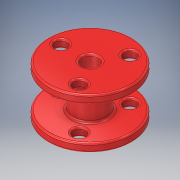
# Autodesk Inventor part: Connecting Rod Hub
Saved by Autodesk Inventor 2017 (Build 210142000, 142)
## iProperties
Created: 2020-01-12
Part Number: Connecting Rod Hub
Material: Stainless Steel
Document SubType Name: Modeling
Designer: Admin
Density: 8 g/cm^3
Appearance: Light Red
Mass: 5.65044 g
Surface Area: 10.6206 cm^2
Volume: 0.706304 cm^3
Author: Admin
Autodesk Inventor part; units mm, degrees
ref_plane "YZ Plane" through (0, 0, 0) normal (1, 0, 0) x (0, 1, 0)
ref_plane "XZ Plane" through (0, 0, 0) normal (0, 1, 0) x (-1, 0, 0)
ref_plane "XY Plane" through (0, 0, 0) normal (0, 0, 1) x (1, 0, 0)
sketch "Sketch1" plane through (0, 0, 0) normal (0, 1, 0) x (-1, 0, 0)
  circle A0 centre (0, 0) radius 3.175
  dimension "d0" = 6.35
  constraints: 1 centre point, 1 coincident
  measures "d0" diameter of A0
extrude "Extrusion1" add sketch "Sketch1" along normal mid plane 6.35
sketch "Sketch2" plane through (0, 3.175, 0) normal (0, 1, 0) x (1, 0, 0)
  circle A0 centre (0, 0) radius 7.9375
  dimension "d3" = 15.875
  constraints: 1 centre point, 1 coincident
  measures "d3" diameter of A0
extrude "Extrusion2" add sketch "Sketch2" along normal blind 1.5875
sketch "Sketch3" plane through (0, -3.175, 0) normal (0, -1, 0) x (1, 0, 0)
  circle A0 centre (0, 0) radius 7.9375
  dimension "d6" = 15.875
  constraints: 1 centre point, 1 coincident
  measures "d6" diameter of A0
extrude "Extrusion3" add sketch "Sketch3" along normal blind 1.5875
sketch "Sketch4" plane through (0, 4.7625, 0) normal (0, 1, 0) x (1, 0, 0)
  circle A0 centre (0, 0) radius 1.5875
  dimension "d9" = 3.175
  constraints: 1 centre point, 1 coincident
  measures "d9" diameter of A0
extrude "Extrusion4" cut sketch "Sketch4" against normal blind 25.4
sketch "Sketch5" plane through (0, 4.7625, 0) normal (0, 1, 0) x (1, 0, 0)
  circle A0 centre (-5.5563, 0) radius 1.1906
  circle A1 centre (2.7781, -4.8119) radius 1.1906
  circle A2 centre (2.7781, 4.8119) radius 1.1906
  point P0 (0, 0)
  dimension "d12" = 2.3813
  dimension "d13" = 0
  dimension "d14" = 5.5563
  dimension "d17" = 360
  constraints: 3 centre point, 7 other
  measures "d12" diameter of A0
  measures "d13" vertical distance of point (0, 0) A0.centre
  measures "d14" distance of point (0, 0) A0.centre
extrude "Extrusion5" cut sketch "Sketch5" against normal blind 25.4
fillet "Fillet1" radius 0.3969 2 edges at (3.175, 3.175, 0) (3.175, -3.175, 0)
fillet "Fillet2" radius 0.3175 18 edges at (-7.9375, 4.7625, 0) (-7.9375, 3.175, 0) (-7.9375, -3.175, 0) (-7.9375, -4.7625, 0) (1.5875, -3.175, 4.8119) (1.5875, -3.175, -4.8119) (1.5875, 4.7625, 4.8119) (-1.5875, 4.7625, 0) (1.5875, 4.7625, -4.8119) (-6.7469, 4.7625, 0) (-6.7469, -3.175, 0) (1.5875, 3.175, 4.8119) (1.5875, 3.175, -4.8119) (-6.7469, 3.175, 0) (1.5875, -4.7625, -4.8119) (-6.7469, -4.7625, 0) (1.5875, -4.7625, 4.8119) (-1.5875, -4.7625, 0)
body "Solid1"
